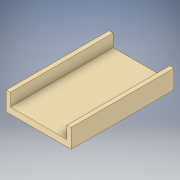
# Autodesk Inventor part: Case_Side
Saved by Autodesk Inventor 2019 (Build 230136000, 136)
## iProperties
Created: 2019-02-21
Part Number: Case_Side
Material: 일반
Document SubType Name: Modeling
Designer: Jeong Ji Hoon
Density: 1 g/cm^3
Appearance: 베이지색
Author: Jeong Ji Hoon
## iProperties of the stored document Case_Side_3D 인쇄.ipt
Created: 2019-02-22
Part Number: Case_Side_3D 인쇄
Material: 일반
Document SubType Name: Modeling
Designer: Jeong Ji Hoon
Density: 1 g/cm^3
Appearance: 기본값
Author: Jeong Ji Hoon
Autodesk Inventor part; units mm, degrees
ref_plane "YZ Plane" through (0, 0, 0) normal (1, 0, 0) x (0, 1, 0)
ref_plane "XZ Plane" through (0, 0, 0) normal (0, 1, 0) x (-1, 0, 0)
ref_plane "XY Plane" through (0, 0, 0) normal (0, 0, 1) x (1, 0, 0)
sketch "스케치1" plane through (0, 0, 0) normal (0, 1, 0) x (-1, 0, 0)
  line L0 (0, 0) -> (15.5, 0)
  line L1 (15.5, 0) -> (15.5, -24.5)
  line L2 (15.5, -24.5) -> (0, -24.5)
  line L3 (0, -24.5) -> (0, 0)
  dimension "d0" = 15.5
  dimension "d1" = 24.5
  constraints: 8 end point, 2 parallel, 1 horizontal, 1 perpendicular
  measures "d0" distance of L1.end L2.end
  measures "d1" distance of L0.end L1.end
extrude "돌출1" add sketch "스케치1" along normal blind 1.5
sketch "스케치2" plane through (0, 1.5, 0) normal (0, 1, 0) x (1, 0, 0)
  line L0 (0, 24.5) -> (-15.5, 24.5) projected
  line L1 (0, 0) -> (-1, 0)
  line L2 (-1, 0) -> (-1, 24.5)
  line L3 (-1, 24.5) -> (0, 24.5)
  line L4 (0, 24.5) -> (0, 0)
  line L5 (-15.5, 0) -> (0, 0) projected
  line L6 (-15.5, 0) -> (-14.5, 0)
  line L7 (-14.5, 0) -> (-14.5, 24.5)
  line L8 (-14.5, 24.5) -> (-15.5, 24.5)
  line L9 (-15.5, 24.5) -> (-15.5, 0)
  dimension "d4" = 1
  dimension "d5" = 1
  constraints: 16 end point, 4 parallel, 2 horizontal, 2 perpendicular, 2 point on line
  measures "d4" distance of L2.end L3.end
  measures "d5" distance of L8.end L7.end
extrude "돌출2" add sketch "스케치2" along normal blind 3 contours L4 L1 L2 L0 | L7 L5 L9 L0
equation "\"d2\" = t"
equation "\"t\" = 1.5"
